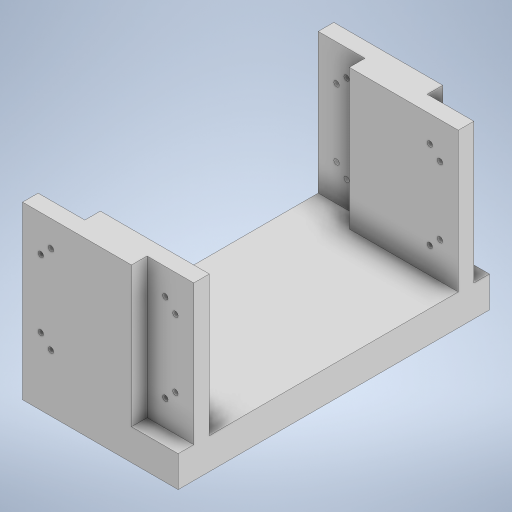
# Autodesk Inventor part: container_mid
Saved by Autodesk Inventor 2023 (Build 270158000, 158)
## iProperties
Created: 2022-11-30
Part Number: container_mid
Material: Genérico
Document SubType Name: Modeling
Designer: inigo
Density: 1 g/cm^3
Appearance: Valor por defecto
Author: inigo
Autodesk Inventor part; units mm, degrees
ref_plane "YZ Plane" through (0, 0, 0) normal (1, 0, 0) x (0, 1, 0)
ref_plane "XZ Plane" through (0, 0, 0) normal (0, 1, 0) x (-1, 0, 0)
ref_plane "XY Plane" through (0, 0, 0) normal (0, 0, 1) x (1, 0, 0)
sketch "Boceto1" plane through (0, 0, 0) normal (0, 0, 1) x (1, 0, 0)
  line L0 (-15, 45) -> (15, 45)
  line L1 (15, 45) -> (15, -45)
  line L2 (15, -45) -> (-15, -45)
  line L3 (-15, -45) -> (-15, 45)
  line L4 (-15, 45) -> (15, -45) construction
  line L5 (15, 45) -> (-15, -45) construction
  point P0 (0, 0)
  dimension "d0" = 30
  dimension "d1" = 90
  constraints: 12 end point, 2 midpoint, 2 parallel, 1 horizontal, 1 perpendicular
  measures "d0" distance of L1.end L2.end
  measures "d1" distance of L0.end L1.end
extrude "Extrusión1" add sketch "Boceto1" along normal blind 10
sketch "Boceto2" plane through (0, 0, 10) normal (0, 0, 1) x (1, 0, 0)
  line L0 (15, 45) -> (15, -45)
  line L1 (5, 30) -> (5, 20)
  line L2 (-5, 30) -> (5, 30)
  line L3 (5, 20) -> (-5, 30) construction
  line L4 (5, 20) -> (-5, 20)
  line L5 (-5, 20) -> (5, 30) construction
  line L6 (-5, 20) -> (-5, 30)
  line L7 (24, 0) -> (9, 0)
  line L8 (-15, -45) -> (15, -45)
  line L9 (5, 25) -> (5.4102, 25)
  circle A0 centre (3.25, 21.75) radius 1.75
  circle A1 centre (-3.25, 28.25) radius 1.75
  line L10 (5, -20) -> (-5, -20)
  circle A2 centre (3.25, -21.75) radius 1.75
  line L11 (5, -25) -> (5.4102, -25)
  line L12 (5, -30) -> (5, -20)
  line L13 (-5, -30) -> (5, -30)
  line L14 (5, -20) -> (-5, -30) construction
  line L15 (-5, -20) -> (5, -30) construction
  line L16 (-5, -20) -> (-5, -30)
  circle A3 centre (-3.25, -28.25) radius 1.75
  line L17 (-15, -45) -> (-15, 45)
  line L18 (15, -45) -> (15, 45) projected
  line L19 (-15, -45) -> (15, -45) projected
  line L20 (-15, 45) -> (15, 45)
  point P0 (0, 0)
  point P1 (-113, 215)
  point P2 (3.25, 28.25)
  point P3 (-3.25, 21.75)
  point P4 (-5, 25)
  point P5 (-3.25, -21.75)
  point P6 (3.25, -28.25)
  point P7 (-143, 115)
  point P8 (-3.25, -21.75)
  point P9 (-5, -25)
  point P10 (3.25, -28.25)
  dimension "d4" = 1.75
  dimension "d5" = 1.75
  dimension "d6" = 1.75
  dimension "d7" = 1.75
  dimension "d8" = 10
  dimension "d9" = 10
  dimension "d10" = 10
  dimension "d11" = 15
  dimension "d12" = 0
  dimension "d13" = 30
  dimension "d14" = 0
  dimension "d15" = 90
  dimension "d16" = 15
  constraints: 34 end point, 15 symmetric about line, 4 centre point, 4 horizontal, 2 midpoint, 2 parallel, 1 perpendicular, 8 other
  measures "d4" distance from line of L2 point (3.25, 28.25)
  measures "d5" distance from line of L1 point (3.25, 28.25)
  measures "d6" distance from line of L6 point (-3.25, 21.75)
  measures "d7" distance from line of L4 point (-3.25, 21.75)
  measures "d8" distance between parallel lines of L4 L2
  measures "d9" distance between parallel lines of L1 L6
  measures "d10" distance between parallel lines of L17 L6
  measures "d12" horizontal extent of L18
  measures "d14" vertical extent of L19
  measures "d16" distance between parallel lines of L20 L2
hole "Agujero1" at (-3.25, 28.25, 10) at (3.25, 21.75, 10) at (3.25, -21.75, 10) at (-3.25, -28.25, 10) direction (0, 0, -1) diameter 3.5 end through all
sketch "Boceto3" plane through (-15, -45, 0) normal (-1, 0, 0) x (0, 0, 1)
  line L0 (0, 0) -> (0, 90) projected
  line L1 (0, 90) -> (20, 90)
  line L2 (20, 90) -> (20, 0)
  line L3 (20, 0) -> (0, 0)
  line L4 (0, 0) -> (0, 90)
  point P0 (0, 45)
  dimension "d24" = 20
  dimension "d25" = 90
  constraints: 8 end point, 2 parallel, 1 horizontal, 1 perpendicular
  measures "d24" distance of L2.end L3.end
  measures "d25" distance of L1.end L2.end
extrude "Extrusión2" add sketch "Boceto3" along normal blind 40
sketch "Boceto4" plane through (-55, -45, 0) normal (-1, 0, 0) x (0, 0, 1)
  line L0 (20, 90) -> (10, 90) projected
  line L1 (10, 0) -> (10, 90) projected
  line L2 (20, 90) -> (10, 90)
  line L3 (10, 90) -> (10, 0)
  line L4 (10, 0) -> (20, 0)
  line L5 (20, 0) -> (20, 90)
  point P0 (0, 45)
  constraints: 8 end point, 2 parallel, 1 horizontal, 1 perpendicular
extrude "Extrusión3" add sketch "Boceto4" along normal blind 30
sketch "Boceto5" plane through (-15, -45, 20) normal (0, 0, 1) x (1, 0, 0)
  line L0 (-40, 0) -> (-40, 90)
  line L1 (-40, 90) -> (-40, 0)
  line L2 (-50, 75) -> (-50, 65)
  line L3 (-60, 75) -> (-50, 75)
  line L4 (-50, 65) -> (-60, 75) construction
  line L5 (-50, 65) -> (-60, 65)
  line L6 (-60, 65) -> (-50, 75) construction
  circle A0 centre (-58.25, 66.75) radius 1.75
  line L7 (-60, 65) -> (-60, 75)
  circle A1 centre (-51.75, 73.25) radius 1.75
  line L8 (-70, -20) -> (-70, 90)
  line L9 (-40, 45) -> (-128, 45)
  line L10 (-50, 25) -> (-60, 25)
  circle A2 centre (-58.25, 23.25) radius 1.75
  line L11 (-50, 15) -> (-50, 25)
  line L12 (-50, 25) -> (-60, 15) construction
  line L13 (-60, 25) -> (-50, 15) construction
  line L14 (-60, 25) -> (-60, 15)
  line L15 (-60, 15) -> (-50, 15)
  circle A3 centre (-51.75, 16.75) radius 1.75
  line L16 (-70, 0) -> (-40, 0)
  line L17 (0, 0) -> (-70, 0) projected
  line L18 (-70, 90) -> (-40, 90)
  line L19 (-70, 0) -> (-70, 90) projected
  point P0 (15, 45)
  point P1 (-60, 70)
  point P2 (-50, 70)
  point P3 (-50, 20)
  point P4 (-60, 20)
  point P5 (-55, 0)
  point P6 (-55, 90)
  dimension "d30" = 3.5
  dimension "d31" = 1.75
  dimension "d32" = 1.75
  dimension "d33" = 1.75
  dimension "d34" = 1.75
  dimension "d35" = 10
  dimension "d36" = 10
  dimension "d38" = 10
  dimension "d39" = 10
  dimension "d40" = 15
  dimension "d41" = 0
  dimension "d42" = 15
  dimension "d43" = 90
  dimension "d45" = 0
  constraints: 36 end point, 8 symmetric about line, 5 midpoint, 4 centre point, 3 equal length, 3 horizontal, 1 perpendicular, 2 other
  measures "d30" diameter of A1
  measures "d31" distance from line of L3 A1.centre
  measures "d32" distance from line of L2 A1.centre
  measures "d33" distance from line of L7 A0.centre
  measures "d34" distance from line of L5 A0.centre
  measures "d35" distance between parallel lines of L5 L3
  measures "d36" distance between parallel lines of L2 L7
  measures "d38" distance between parallel lines of L8 L7
  measures "d39" distance from line of L0 point (-50, 70)
  measures "d40" distance between parallel lines of L16 L15
  measures "d41" distance from line of L17 point (-55, 0)
  measures "d42" distance between parallel lines of L18 L3
  measures "d43" distance from line of L16 point (-55, 90)
  measures "d45" distance between parallel lines of L19 L8
hole "Agujero2" at (-66.75, 28.25, 20) at (-73.25, 21.75, 20) at (-73.25, -21.75, 20) at (-66.75, -28.25, 20) direction (0, 0, -1) diameter 3.5 end through all
sketch "Boceto6" plane through (-15, -45, 20) normal (0, 0, 1) x (1, 0, 0)
  line L0 (-40, 0) -> (-70, 0) projected
  line L1 (-70, 0) -> (30, 0)
  line L2 (30, 0) -> (30, -20)
  line L3 (30, -20) -> (-70, -20)
  line L4 (-70, -20) -> (-70, 0)
  point P0 (15, 45)
  dimension "d53" = 20
  constraints: 8 end point, 2 parallel, 1 horizontal, 1 perpendicular
  measures "d53" distance of L1.end L2.end
extrude "Extrusión4" add sketch "Boceto6" against normal blind 100
mirror "Simetría1" about plane through (-35, -55, -80) normal (0, 0, -1) of "Extrusión1", "Agujero1", "Extrusión2", "Agujero2", "Extrusión3", "Extrusión4"
